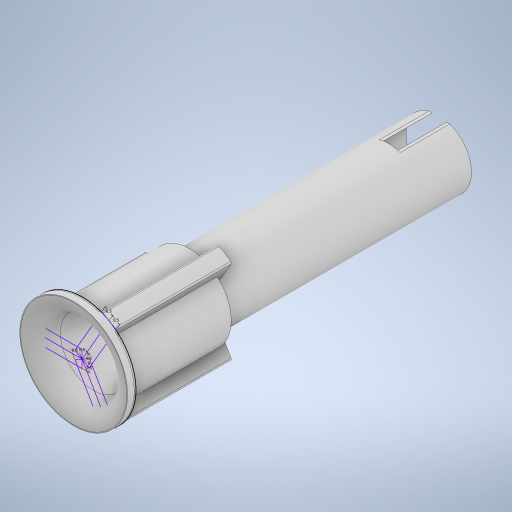
# Autodesk Inventor part: 內部按鈕(下)
Saved by Autodesk Inventor 2024.2 (Build 282272000, 272)
## iProperties
Created: 2024-04-18
Part Number: 內部按鈕(下)
Material: 一般
Document SubType Name: Modeling
Designer: User
Density: 1 g/cm^3
Appearance: 預設
Author: User
Autodesk Inventor part; units mm, degrees
ref_plane "YZ Plane" through (0, 0, 0) normal (1, 0, 0) x (0, 1, 0)
ref_plane "XZ Plane" through (0, 0, 0) normal (0, 1, 0) x (-1, 0, 0)
ref_plane "XY Plane" through (0, 0, 0) normal (0, 0, 1) x (1, 0, 0)
sketch "草圖1" plane through (0, 0, 0) normal (0, 1, 0) x (-1, 0, 0)
  line L0 (0, 0) -> (0, -15)
  line L1 (0, -15) -> (2, -15)
  line L2 (2, -15) -> (2, 0)
  line L3 (2, 0) -> (0, 0)
  dimension "d0" = 15
  dimension "d1" = 2
  constraints: 8 end point, 2 parallel, 1 perpendicular, 1 vertical
  measures "d0" distance of L0.start L0.end
  measures "d1" distance of L1.end L0.end
revolve "迴轉1" add sketch "草圖1" angle 360 about axis through (0, 0, 0) along (0, 0, -1)
sketch "草圖2" plane through (0, 0, 0) normal (0, 0, 1) x (1, 0, 0)
  circle A0 centre (0, 0) radius 2.5
  dimension "d3" = 5
  constraints: 1 centre point, 1 coincident
  measures "d3" diameter of A0
extrude "擠出1" add sketch "草圖2" along normal blind 7
sketch "草圖3" plane through (0, 0, 7) normal (0, 0, 1) x (1, 0, 0)
  circle A0 centre (0, 0) radius 3.25
  dimension "d6" = 6.5
  constraints: 1 centre point, 1 coincident
  measures "d6" diameter of A0
extrude "擠出2" add sketch "草圖3" against normal blind 0.5
sketch "草圖4" plane through (0, 0, 6.5) normal (0, 0, -1) x (-1, 0, 0)
  circle A0 centre (0, 0) radius 3.25 projected
  line L0 (0, 0) -> (0, -0.5)
  line L1 (0, -0.5) -> (3.25, -0.5)
  line L2 (3.25, -0.5) -> (3.25, 0)
  line L3 (3.25, 0) -> (0, 0)
  line L4 (0, 0) -> (0, 0.5)
  line L5 (0, 0.5) -> (3.25, 0.5)
  line L6 (3.25, 0.5) -> (3.25, 0)
  circle A1 centre (0, 0) radius 2.5 projected
  line L7 (0, 0) -> (0.433, -0.25)
  line L8 (0.433, -0.25) -> (-1.192, -3.0646)
  line L9 (-1.192, -3.0646) -> (-1.625, -2.8146)
  line L10 (-1.625, -2.8146) -> (0, 0)
  line L11 (0, 0) -> (-0.433, 0.25)
  line L12 (-0.433, 0.25) -> (-2.058, -2.5646)
  line L13 (-2.058, -2.5646) -> (-1.625, -2.8146)
  line L14 (-1.625, 2.8146) -> (-2.058, 2.5646)
  line L15 (-2.058, 2.5646) -> (-0.433, -0.25)
  line L16 (-0.433, -0.25) -> (0, 0)
  line L17 (0, 0) -> (-1.625, 2.8146)
  line L18 (-1.625, 2.8146) -> (-1.192, 3.0646)
  line L19 (-1.192, 3.0646) -> (0.433, 0.25)
  line L20 (0.433, 0.25) -> (0, 0)
  circle A2 centre (0, 0) radius 2.5
  circle A3 centre (0, 0) radius 3.25
  point P0 (-0.7917, 2.3713)
  point P1 (-1.1726, 3.0311)
  point P2 (-2.0387, 2.5311)
  point P3 (-1.6578, 1.8713)
  point P4 (-1.1726, -3.0311)
  point P5 (-0.7917, -2.3713)
  point P6 (-1.6578, -1.8713)
  point P7 (-2.0387, -2.5311)
  point P8 (2.4495, 0.5)
  point P9 (2.4495, -0.5)
  point P10 (3.2113, -0.5)
  point P11 (3.2113, 0.5)
  point P12 (0.2887, 0.5)
  point P13 (-1.25, 2.1651)
  point P14 (0.2887, -0.5)
  point P15 (2.5, 0)
  point P16 (-1.25, -2.1651)
  point P17 (-0.5774, 0)
  dimension "d10" = 0.5
  dimension "d11" = 0.5
  dimension "d12" = 0.5
  dimension "d13" = 0.5
  dimension "d14" = 0.5
  dimension "d15" = 0.5
  constraints: 42 end point, 9 parallel, 5 perpendicular, 3 coincident, 2 centre point, 1 concentric, 7 other
  measures "d10" distance of L0.end L0.start
  measures "d11" distance of L0.start L4.end
  measures "d12" distance of L7.start L7.end
  measures "d13" distance of L11.end L7.start
  measures "d14" distance of L14.end L14.start
  measures "d15" distance of L14.start L18.end
extrude "擠出3" add sketch "草圖4" along normal blind 7 contours L3 A1 L5 A0 | A0 L1 A1 L3 | A1 L1 L8 L7 L3 | L3 L20 L19 L5 A1 | L19 A1 L17 A0 | A0 L10 A1 L8 | L17 A1 L19 L5 L4 | L0 L1 L8 A1 L10 | L10 A1 L12 L15 L16 | L11 L12 L15 A1 L17 | L17 A1 L15 A0 | A0 L12 A1 L10
fillet "圓角1" radius 0.2 10 edges at (-1.25, -2.1651, 6.5) (2.2797, -1.0261, 6.5) (2.2797, 1.0261, 6.5) (-2.8304, -0.5, 6.5) (0.9822, -2.7012, 6.5) (1.8482, -2.2012, 6.5) (1.8482, 2.2012, 6.5) (-1.25, 2.1651, 6.5) (0.9822, 2.7012, 6.5) (-2.8304, 0.5, 6.5)
fillet "圓角2" radius 0.15 3 edges at (-1, 1.7321, 0) (-1, -1.7321, 0) (2, 0, 0)
sketch "草圖5" plane through (0, 0, 7) normal (0, 0, 1) x (1, 0, 0)
  point P0 (0, 0)
  point P1 (0, 0)
  constraints: 1 coincident
hole "孔1" at (0, 0, 7) direction (0, 0, -1) diameter 4 depth 6 tip angle 118
fillet "圓角3" radius 1.2 1 edges at (0, 2, 7)
fillet "圓角4" radius 0.1 16 edges at (1.1175, 3.0518, 6.4409) (1.1726, 3.0311, 2.9) (-3.2017, 0.5581, 6.4409) (-3.2113, 0.5, 2.9) (-1.625, 2.8146, 6.5) (-3.2017, -0.5581, 6.4409) (-3.2113, -0.5, 2.9) (1.1175, -3.0518, 6.4409) (1.1726, -3.0311, 2.9) (-1.625, -2.8146, 6.5) (2.0842, -2.4937, 6.4409) (2.0387, -2.5311, 2.9) (2.0842, 2.4937, 6.4409) (2.0387, 2.5311, 2.9) (2.9741, -1.3105, 6.5) (2.9741, 1.3105, 6.5)
sketch "草圖6" plane through (0, 0, -15) normal (0, 0, -1) x (-1, 0, 0)
  circle A0 centre (0, 0) radius 2 projected
  line L0 (0, -2) -> (-1.5, -2)
  line L1 (-1.5, -2) -> (-1.5, -1.9)
  line L2 (-1.5, -1.9) -> (0, -1.9)
  line L3 (0, -1.9) -> (0, -2)
  line L4 (0, -2) -> (0, -1.9)
  line L5 (0, -1.9) -> (1.5, -1.9)
  line L6 (1.5, -1.9) -> (1.5, -2)
  line L7 (1.5, -2) -> (0, -2)
  line L8 (-1.4991, 1.9473) -> (-1.4956, 1.8474)
  line L9 (-1.4956, 1.8474) -> (0.0035, 1.9001)
  line L10 (0.0035, 1.9001) -> (0, 2)
  line L11 (0.0035, 1.9001) -> (0, 2)
  line L12 (1.4991, 2.0527) -> (1.5026, 1.9528)
  line L13 (1.5026, 1.9528) -> (0.0035, 1.9001)
  line L14 (-1.4991, 1.9473) -> (-1.4991, 2.0527)
  line L15 (-1.4991, 2.0527) -> (1.4954, 2.158)
  line L16 (1.4954, 2.158) -> (1.5018, 1.975)
  dimension "d31" = 1.5
  dimension "d32" = 0.1
  dimension "d33" = 1.5
  dimension "d34" = 1.5
  dimension "d35" = 0.1
  dimension "d36" = 1.5
  constraints: 34 end point, 7 equal length, 2 perpendicular, 2 point on circle, 2 point on line, 2 vertical, 1 horizontal, 1 tangent
  measures "d31" distance of L0.start L0.end
  measures "d32" distance of L0.end L1.end
  measures "d33" distance of L2.end L5.end
  measures "d34" distance of L10.end L8.start
  measures "d35" distance of L8.end L8.start
  measures "d36" distance of L10.end L12.start
extrude "擠出5" cut sketch "草圖6" against normal blind 3 contours L13 L10 A0 | A0 L9 L8 L14 L15 L16 L12 L13 | L5 L6 L7 A0 | A0 L3 L5 | L10 L9 A0 | L0 L1 L2 A0 | A0 L2 L3
sketch "草圖7" plane through (0.6245, -1.9, -15) normal (0, 0, -1) x (-1, 0, 0)
  circle A0 centre (0.6245, 1.9) radius 1.95
  dimension "d39" = 3.9
  constraints: 1 centre point, 1 coincident
  measures "d39" diameter of A0
extrude "擠出7" cut sketch "草圖7" against normal blind 3
sketch "草圖8" plane through (-0.4387, -1.9, -15) normal (0, 0, -1) x (-1, 0, 0)
  circle A0 centre (-0.4387, 1.9) radius 0.5
  dimension "d44" = 1
  constraints: 1 centre point, 1 coincident
  measures "d44" diameter of A0
extrude "擠出9" cut sketch "草圖8" against normal blind 15
